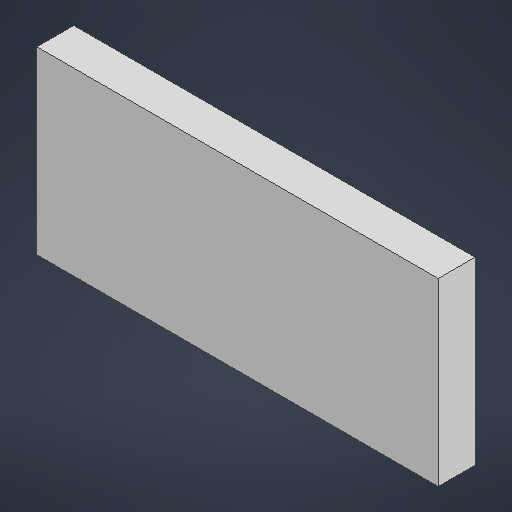
# Autodesk Inventor part: motor_bracket_base
Saved by Autodesk Inventor 2026 (Build 300175050, 175E)
## iProperties
Created: 2025-11-11
Part Number: motor_bracket_base
Material: Generic
Document SubType Name: Modeling
Designer: habbo
Density: 1 g/cm^3
Appearance: Default
Author: habbo
Autodesk Inventor part; units mm, degrees
ref_plane "YZ Plane" through (0, 0, 0) normal (1, 0, 0) x (0, 1, 0)
ref_plane "XZ Plane" through (0, 0, 0) normal (0, 1, 0) x (-1, 0, 0)
ref_plane "XY Plane" through (0, 0, 0) normal (0, 0, 1) x (1, 0, 0)
sketch "Sketch1" plane through (0, 0, 0) normal (0, 0, 1) x (1, 0, 0)
  line L0 (-44.55, -20) -> (44.55, -20)
  line L1 (44.55, -20) -> (44.55, 20)
  line L2 (44.55, 20) -> (-44.55, 20)
  line L3 (-44.55, 20) -> (-44.55, -20)
  line L4 (-44.55, -20) -> (44.55, 20) construction
  line L5 (44.55, -20) -> (-44.55, 20) construction
  point P0 (0, 0)
  dimension "d0" = 89.1
  dimension "d1" = 40
  constraints: 12 end point, 2 midpoint, 2 parallel, 1 horizontal, 1 perpendicular
  measures "d0" distance of L2.end L1.end
  measures "d1" distance of L1.end L0.end
extrude "Extrusion1" add sketch "Sketch1" along normal mid plane 8.193
body "Solid1"
